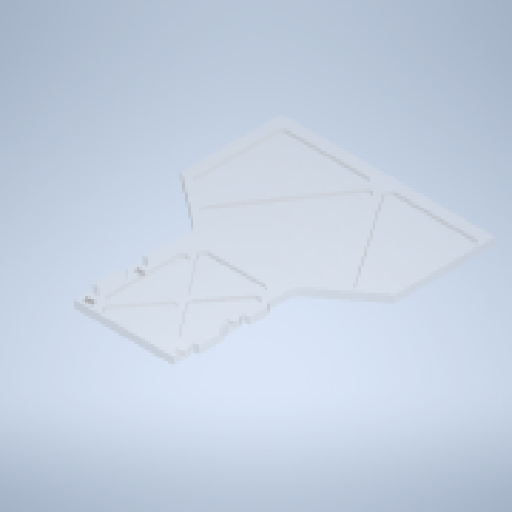
# Autodesk Inventor part: new_hera
Saved by Autodesk Inventor 2024 (Build 280153000, 153)
## iProperties
Created: 2023-12-17
Part Number: new_hera
Material: ポリカーボネート、クリア
Document SubType Name: Modeling
Designer: right
Density: 1.2 g/cm^3
Appearance: ポリカーボネート - クリア
Mass: 15.0866 g
Surface Area: 150.969 cm^2
Volume: 12.5721 cm^3
Author: right
Autodesk Inventor part; units mm, degrees
ref_plane "YZ Plane" through (0, 0, 0) normal (1, 0, 0) x (0, 1, 0)
ref_plane "XZ Plane" through (0, 0, 0) normal (0, 1, 0) x (-1, 0, 0)
ref_plane "XY Plane" through (0, 0, 0) normal (0, 0, 1) x (1, 0, 0)
sketch "スケッチ1" plane through (0, 0, 0) normal (0, 1, 0) x (-1, 0, 0)
  line L0 (-19.75, 24) -> (19.75, 24)
  line L1 (19.75, 24) -> (19.75, -24)
  line L2 (19.75, -24) -> (-19.75, -24)
  line L3 (-19.75, -24) -> (-19.75, 24)
  line L4 (-19.75, 24) -> (19.75, -24) construction
  line L5 (19.75, 24) -> (-19.75, -24) construction
  line L6 (19.75, 0) -> (-19.75, 0) construction
  line L7 (-19.75, 0) -> (19.75, -24) construction
  line L8 (19.75, 0) -> (-19.75, -24) construction
  line L9 (21.25, 15) -> (-21.25, 15)
  line L10 (-21.25, 15) -> (-21.25, 5)
  line L11 (-21.25, 5) -> (21.25, 5)
  line L12 (21.25, 5) -> (21.25, 15)
  line L13 (21.25, 15) -> (-21.25, 5) construction
  line L14 (-21.25, 15) -> (21.25, 5) construction
  circle A0 centre (19.75, 3.9) radius 1.1
  line L15 (0, 5) -> (0, 10) construction
  line L16 (21.25, 10) -> (0, 10) construction
  circle A1 centre (19.75, 16.1) radius 1.1
  circle A2 centre (-19.75, 3.9) radius 1.1
  circle A3 centre (-19.75, 16.1) radius 1.1
  line L17 (21.25, -15) -> (-21.25, -15)
  line L18 (-21.25, -15) -> (-21.25, -5)
  line L19 (-21.25, -5) -> (21.25, -5)
  line L20 (21.25, -5) -> (21.25, -15)
  line L21 (21.25, -15) -> (-21.25, -5) construction
  line L22 (-21.25, -15) -> (21.25, -5) construction
  circle A4 centre (19.75, -3.9) radius 1.1
  line L23 (0, -5) -> (0, -10) construction
  line L24 (21.25, -10) -> (0, -10) construction
  circle A5 centre (19.75, -16.1) radius 1.1
  circle A6 centre (-19.75, -16.1) radius 1.1
  circle A7 centre (-19.75, -3.9) radius 1.1
  point P0 (0, 0)
  point P1 (-19.75, 17.2)
  point P2 (-19.75, 15)
  point P3 (-19.75, 5)
  point P4 (-19.75, 2.8)
  point P5 (-19.75, -2.8)
  point P6 (-19.75, -5)
  point P7 (-19.75, -15)
  point P8 (-19.75, -17.2)
  point P9 (19.75, -17.2)
  point P10 (19.75, -15)
  point P11 (19.75, -5)
  point P12 (19.75, -2.8)
  point P13 (19.75, 2.8)
  point P14 (19.75, 5)
  point P15 (19.75, 15)
  point P16 (19.75, 17.2)
  point P17 (19.75, -15)
  point P18 (-19.75, -15)
  dimension "d1" = 48
  dimension "d2" = 39.5
  dimension "d3" = 10
  dimension "d4" = 1.5
  dimension "d5" = 2.2
  dimension "d6" = 10
  dimension "d7" = 1.5
  constraints: 50 end point, 14 symmetric about line, 8 centre point, 8 midpoint, 4 parallel, 3 perpendicular, 2 horizontal, 1 point on line, 1 tangent, 1 vertical, 7 other
  measures "d1" distance of L2.end L0.start
  measures "d2" distance between parallel lines of L3 L1
  measures "d3" distance of L10.end L9.end
  measures "d4" distance between parallel lines of L3 L10
  measures "d5" diameter of A0
  measures "d6" distance between parallel lines of L19 L11
  measures "d7" distance between parallel lines of L1 L12
extrude "押し出し1" add sketch "スケッチ1" along normal blind 3 contours L0 L1 A1 L9 A3 L3 | L9 L1 L11 L3 | L3 L11 L10 L9 | L9 L12 L11 L1 | L11 A0 L1 A4 L19 A7 L3 A2 | L19 L1 L17 L3 | L3 L17 L18 L19 | L19 L20 L17 L1 | A6 L3 | L17 A5 L1 L2 L3 A6 | L1 A5 picked at (-19.4196, -15.9409) picked at (19.6623, -16.456)
sketch "スケッチ2" plane through (-19.75, 0, 17.2) normal (-1, 0, 0) x (0, 0, 1)
  line L0 (6.8, 0) -> (6.8, 3) construction
  line L1 (6.8, 1.5) -> (-41.2, 1.5) construction
  line L2 (-41.2, 0) -> (-41.2, 3) construction
  line L3 (-2.2, 3) -> (-12.2, 3) construction
  line L4 (-7.2, 3) -> (-7.2, 0) construction
  line L5 (-12.2, 0) -> (-12.2, 3) construction
  point P0 (-17.2, 0)
  point P1 (-17.2, 1.5)
  point P2 (2.8, 1.5)
  dimension "d10" = 5
  constraints: 4 end point, 4 midpoint, 1 symmetric about line, 1 vertical
  measures "d10" distance from line of L5 point (-17.2, 1.5)
hole "穴1" at (-19.75, 1.5, 0) at (-19.75, 1.5, 20) direction (1, 0, 0) diameter 1.567 end through all thread size "M2x0.4" class "6H" standard "ISO Metric profile"
sketch "スケッチ3" plane through (0, 3, 0) normal (0, 1, 0) x (1, 0, 0)
  line L0 (42.5, 81.5) -> (-42.5, 81.5)
  line L1 (19.75, 24) -> (-19.75, 24) projected
  circle A0 centre (0, -173.5) radius 4 projected
  line L2 (0, 81.5) -> (0, 24) construction
  line L3 (42.5, 81.5) -> (42.5, 41.5)
  line L4 (42.5, 41.5) -> (19.75, 24)
  line L5 (-42.5, 41.5) -> (-19.75, 24)
  line L6 (-42.5, 81.5) -> (-42.5, 41.5)
  point P0 (0, 0)
  dimension "d18" = 255
  dimension "d19" = 85
  dimension "d20" = 40
  constraints: 12 end point, 2 midpoint, 2 vertical, 1 horizontal, 1 symmetric about line, 1 vertical alignment
  measures "d18" distance from line of A0.centre L0
  measures "d19" distance of L0.start L0.end
  measures "d20" distance of L0.start L3.end
extrude "押し出し2" add sketch "スケッチ3" against normal up to surface (3 mm away) contours L3 L4 L1 L5 L6 L0
fillet "フィレット1" radius 5.75 2 edges at (-19.75, 1.5, -24) (19.75, 1.5, -24)
sketch "スケッチ6" plane through (0, 3, 0) normal (0, 1, 0) x (1, 0, 0)
  arc A0 (19.75, 15) -> (21.3608, 12.8804) centre (21.95, 15) ccw
  line L0 (19.75, 15) -> (19.75, 21.1687) projected
  line L1 (21.25, 14) -> (21.25, -21.2075)
  line L2 (21.25, 18) -> (21.25, 14)
  line L3 (21.25, 15) -> (19.75, 15) projected
  line L4 (0, 0) -> (0, -24) construction
  line L5 (-19.75, -24) -> (19.75, -24) construction
  arc A1 (-21.3608, 12.8804) -> (-19.75, 15) centre (-21.95, 15) ccw
  line L6 (-21.25, 15) -> (-19.75, 15)
  line L7 (-21.25, 14) -> (-21.25, 18)
  line L8 (-21.25, 14) -> (-21.25, -21.2075)
  point P0 (21.25, 12.9143)
  point P1 (-21.25, 12.9143)
  dimension "d30" = 2.2
  constraints: 12 end point, 5 symmetric about line, 4 point on circle, 4 vertical, 2 centre point, 1 midpoint, 1 tangent, 7 other
  measures "d30" radius of A0
extrude "押し出し4" cut sketch "スケッチ6" against normal through all
sketch "スケッチ7" plane through (0, 0, 0) normal (0, -1, 0) x (1, 0, 0)
  line L0 (-19.75, -21.1687) -> (-19.75, -15) projected
  line L1 (19.75, -15) -> (19.75, -21.1687) projected
  line L2 (-19.75, -15) -> (19.75, -15)
  line L3 (-21.9942, -25.7263) -> (-42.5, -41.5) projected
  arc A0 (-21.9942, -25.7263) -> (-19.75, -21.1687) centre (-25.5, -21.1687) ccw projected
  line L4 (-42.5, -41.5) -> (-42.5, -81.5) projected
  line L5 (-42.5, -81.5) -> (42.5, -81.5) projected
  arc A1 (19.75, -21.1687) -> (21.9942, -25.7263) centre (25.5, -21.1687) ccw projected
  line L6 (42.5, -41.5) -> (21.9942, -25.7263) projected
  line L7 (42.5, -81.5) -> (42.5, -41.5) projected
  line L8 (-16.75, -21.1687) -> (-16.75, -18)
  line L9 (-16.75, -18) -> (16.75, -18)
  line L10 (16.75, -18) -> (16.75, -21.1687)
  arc A2 (16.75, -21.1687) -> (20.165, -28.1042) centre (25.5, -21.1687) ccw
  line L11 (20.165, -28.1042) -> (39.5, -42.9772)
  line L12 (39.5, -42.9772) -> (39.5, -78.5)
  line L13 (39.5, -78.5) -> (-39.5, -78.5)
  line L14 (-39.5, -78.5) -> (-39.5, -42.9772)
  line L15 (-39.5, -42.9772) -> (-20.165, -28.1042)
  arc A3 (-20.165, -28.1042) -> (-16.75, -21.1687) centre (-25.5, -21.1687) ccw
  line L16 (0, -78.5) -> (-29.8325, -35.5407) construction
  line L17 (0, -78.5) -> (29.8325, -35.5407) construction
  line L18 (0, -78.5) -> (0, -18) construction
  line L19 (1.1903, -77.5843) -> (-28.5587, -34.7452)
  line L20 (-28.5587, -34.7452) -> (-31.0229, -36.4563)
  line L21 (-31.0229, -36.4563) -> (-1.2738, -79.2955)
  line L22 (-1.2738, -79.2955) -> (1.1903, -77.5843)
  line L23 (1.1903, -77.5843) -> (-31.0229, -36.4563) construction
  line L24 (-28.5587, -34.7452) -> (-1.2738, -79.2955) construction
  line L25 (-1.1903, -77.5843) -> (28.6422, -34.625)
  line L26 (31.0229, -36.4563) -> (1.2738, -79.2955)
  line L27 (20.165, -28.1042) -> (-20.165, -28.1042)
  line L28 (-20.165, -28.1042) -> (-20.165, -25.1042)
  line L29 (-20.165, -25.1042) -> (20.165, -25.1042)
  line L30 (20.165, -25.1042) -> (20.165, -28.1042)
  line L31 (-28.5587, -34.7452) -> (-28.6355, -34.6199)
  point P0 (0, 0)
  point P1 (-14.9163, -57.0203)
  point P2 (28.5587, -34.7452)
  point P3 (31.0229, -36.4563)
  point P4 (-29.2396, -35.4437)
  point P5 (-1.8262, -78.5)
  point P6 (-31.7065, -37.1534)
  point P7 (0, -75.8702)
  point P8 (29.2396, -35.4437)
  point P9 (1.8262, -78.5)
  point P10 (-17.685, -25.1042)
  point P11 (17.685, -25.1042)
  point P12 (-0.1282, -78.5)
  point P13 (-19.5553, -28.8968)
  point P14 (-19.5553, -28.8968)
  dimension "d33" = 3
  dimension "d34" = 3
  dimension "d38" = 3
  constraints: 50 end point, 8 point on line, 7 midpoint, 5 parallel, 4 point on circle, 4 symmetric about line, 2 centre point, 2 horizontal, 2 perpendicular, 9 other
  measures "d33" radial gap between concentric circles of A0 A3
  measures "d34" distance of L20.end L19.end
  measures "d38" distance between parallel lines of L27 L29
extrude "押し出し5" cut sketch "スケッチ7" against normal blind 1.5 contours L27 L11 L25 L19 L31 L15 | L21 L13 L14 L15 | L11 L12 L13 L26
fillet "フィレット3" radius 2 14 edges at (0, 0.75, -75.8702) (1.8262, 0.75, -78.5) (-1.8262, 0.75, -78.5) (31.0229, 0.75, -36.4563) (39.5, 0.75, -78.5) (39.5, 0.75, -42.9772) (-39.5, 0.75, -42.9772) (-39.5, 0.75, -78.5) (-31.0229, 0.75, -36.4563) (-20.165, 0.75, -28.1042) (20.165, 0.75, -28.1042) (28.6422, 0.75, -34.625) (-28.6355, 0.75, -34.6199) (-28.5587, 0.75, -34.7452)
sketch "スケッチ8" plane through (0, 0, 0) normal (0, -1, 0) x (1, 0, 0)
  line L0 (19.75, 20.7835) -> (-19.75, 20.7835) projected
  line L1 (-10.771, -20.7835) -> (10.771, -20.7835)
  line L2 (16.25, -13.479) -> (16.25, 13.479)
  line L3 (10.771, 20.7835) -> (-10.771, 20.7835)
  line L4 (-16.25, 13.479) -> (-16.25, -13.479)
  line L5 (-16.25, -20.7835) -> (16.25, 20.7835) construction
  line L6 (16.25, -20.7835) -> (-16.25, 20.7835) construction
  line L7 (-21.25, 5) -> (-21.25, 15) projected
  arc A0 (-14.25, 20.7835) -> (-16.25, 18.7835) centre (-14.25, 18.7835) ccw
  arc A1 (16.25, 18.7835) -> (14.25, 20.7835) centre (14.25, 18.7835) ccw
  arc A2 (14.25, -20.7835) -> (16.25, -18.7835) centre (14.25, -18.7835) ccw
  arc A3 (-16.25, -18.7835) -> (-14.25, -20.7835) centre (-14.25, -18.7835) ccw
  line L8 (12.3514, -17.5578) -> (-12.6696, 14.7046)
  line L9 (-16.4544, 19.5849) -> (-14.874, 20.8106)
  line L10 (-12.3514, 17.5578) -> (12.6696, -14.7046)
  line L11 (16.4544, -19.5849) -> (14.874, -20.8106)
  line L12 (14.874, -20.8106) -> (-14.874, 20.8106) construction
  line L13 (-16.4544, 19.5849) -> (16.4544, -19.5849) construction
  arc A4 (-12.6696, 14.7046) -> (-16.25, 13.479) centre (-14.25, 13.479) ccw
  arc A5 (-10.771, 20.7835) -> (-12.3514, 17.5578) centre (-10.771, 18.7835) ccw
  arc A6 (12.6696, -14.7046) -> (16.25, -13.479) centre (14.25, -13.479) ccw
  arc A7 (10.771, -20.7835) -> (12.3514, -17.5578) centre (10.771, -18.7835) ccw
  line L14 (0, 0) -> (0, 20.7835) construction
  line L15 (-12.3514, -17.5578) -> (12.6696, 14.7046)
  line L16 (12.3514, 17.5578) -> (-12.6696, -14.7046)
  arc A8 (12.3514, 17.5578) -> (10.771, 20.7835) centre (10.771, 18.7835) ccw
  arc A9 (16.25, 13.479) -> (12.6696, 14.7046) centre (14.25, 13.479) ccw
  arc A10 (-12.3514, -17.5578) -> (-10.771, -20.7835) centre (-10.771, -18.7835) ccw
  arc A11 (-16.25, -13.479) -> (-12.6696, -14.7046) centre (-14.25, -13.479) ccw
  point P0 (-15.6642, 20.1977)
  point P1 (12.6696, 14.7046)
  point P2 (12.3514, 17.5578)
  point P3 (-12.6696, -14.7046)
  point P4 (-12.3514, -17.5578)
  point P5 (0, 1.6317)
  point P6 (1.2655, 0)
  point P7 (0, -1.6317)
  point P8 (-1.2655, 0)
  dimension "d39" = 5
  dimension "d40" = 2
  dimension "d41" = 2
  dimension "d42" = 2
  dimension "d43" = 2
  constraints: 30 end point, 25 point on circle, 25 point on line, 24 tangent, 12 centre point, 9 equal radius, 6 midpoint, 4 parallel, 4 symmetric about line, 3 perpendicular, 1 horizontal
  measures "d39" distance between parallel lines of L7 L4
  measures "d40" radius of A0
  measures "d41" distance between parallel lines of L8 L10
  measures "d42" radius of A4
  measures "d43" radius of A8
extrude "押し出し6" cut sketch "スケッチ8" against normal blind 1.5 contours A8 L16 L10 A5 L0 | L15 A9 L2 A6 L10 | L8 A7 L1 A10 L15 | L16 A11 L4 A4 L8
sketch "スケッチ9" plane through (0, 1.5, 0) normal (0, -1, 0) x (1, 0, 0)
  line L0 (12.6696, -14.7046) -> (1.2655, 0) projected
  line L1 (1.2655, 0) -> (12.6696, 14.7046) projected
  arc A0 (16.25, 13.479) -> (12.6696, 14.7046) centre (14.25, 13.479) ccw projected
  line L2 (16.25, 13.479) -> (16.25, -13.479) projected
  arc A1 (12.6696, -14.7046) -> (16.25, -13.479) centre (14.25, -13.479) ccw projected
  line L3 (-12.3514, -17.5578) -> (0, -1.6317) projected
  line L4 (0, -1.6317) -> (12.3514, -17.5578) projected
  arc A2 (10.771, -20.7835) -> (12.3514, -17.5578) centre (10.771, -18.7835) ccw projected
  line L5 (10.771, -20.7835) -> (-10.771, -20.7835) projected
  arc A3 (-12.3514, -17.5578) -> (-10.771, -20.7835) centre (-10.771, -18.7835) ccw projected
  arc A4 (-10.771, 20.7835) -> (-12.3514, 17.5578) centre (-10.771, 18.7835) ccw projected
  line L6 (-10.771, 20.7835) -> (10.771, 20.7835) projected
  arc A5 (12.3514, 17.5578) -> (10.771, 20.7835) centre (10.771, 18.7835) ccw projected
  line L7 (12.3514, 17.5578) -> (0, 1.6317) projected
  line L8 (0, 1.6317) -> (-12.3514, 17.5578) projected
  line L9 (-12.6696, 14.7046) -> (-1.2655, 0) projected
  line L10 (-1.2655, 0) -> (-12.6696, -14.7046) projected
  arc A6 (-16.25, -13.479) -> (-12.6696, -14.7046) centre (-14.25, -13.479) ccw projected
  line L11 (-16.25, -13.479) -> (-16.25, 13.479) projected
  arc A7 (-12.6696, 14.7046) -> (-16.25, 13.479) centre (-14.25, 13.479) ccw projected
  line L12 (-29.8251, -38.1811) -> (-4.0073, -75.3592) projected
  arc A8 (-5.65, -78.5) -> (-4.0073, -75.3592) centre (-5.65, -76.5) ccw projected
  line L13 (-5.65, -78.5) -> (-37.5, -78.5) projected
  arc A9 (-39.5, -76.5) -> (-37.5, -78.5) centre (-37.5, -76.5) ccw projected
  line L14 (-39.5, -76.5) -> (-39.5, -43.962) projected
  arc A10 (-38.7194, -42.3768) -> (-39.5, -43.962) centre (-37.5, -43.962) ccw projected
  line L15 (-38.7194, -42.3768) -> (-32.6873, -37.7366) projected
  arc A11 (-29.8251, -38.1811) -> (-32.6873, -37.7366) centre (-31.4679, -39.3219) ccw projected
  line L16 (4.0073, -75.3592) -> (29.8251, -38.1811) projected
  arc A12 (32.6873, -37.7366) -> (29.8251, -38.1811) centre (31.4679, -39.3219) ccw projected
  line L17 (32.6873, -37.7366) -> (38.7194, -42.3768) projected
  arc A13 (39.5, -43.962) -> (38.7194, -42.3768) centre (37.5, -43.962) ccw projected
  line L18 (39.5, -43.962) -> (39.5, -76.5) projected
  arc A14 (37.5, -78.5) -> (39.5, -76.5) centre (37.5, -76.5) ccw projected
  line L19 (37.5, -78.5) -> (5.65, -78.5) projected
  arc A15 (4.0073, -75.3592) -> (5.65, -78.5) centre (5.65, -76.5) ccw projected
  line L20 (-27.1323, -33.4636) -> (-20.7042, -28.5189) projected
  arc A16 (-19.4848, -28.1042) -> (-20.7042, -28.5189) centre (-19.4848, -30.1042) ccw projected
  line L21 (-19.4848, -28.1042) -> (19.4848, -28.1042) projected
  arc A17 (20.7042, -28.5189) -> (19.4848, -28.1042) centre (19.4848, -30.1042) ccw projected
  line L22 (20.7042, -28.5189) -> (27.1323, -33.4636) projected
  arc A18 (27.5556, -36.1896) -> (27.1323, -33.4636) centre (25.9129, -35.0489) ccw projected
  line L23 (27.5556, -36.1896) -> (1.6427, -73.5046) projected
  arc A19 (-1.6427, -73.5046) -> (1.6427, -73.5046) centre (0, -72.3639) ccw projected
  line L24 (-1.6427, -73.5046) -> (-27.5556, -36.1896) projected
  arc A20 (-27.1323, -33.4636) -> (-27.5556, -36.1896) centre (-25.9129, -35.0489) ccw projected
  arc A21 (21.25, -12.9143) -> (19.75, -15) centre (21.95, -15) ccw projected
  line L25 (21.25, -5) -> (21.25, -12.9143) projected
  line L26 (19.75, -5) -> (21.25, -5) projected
  arc A22 (19.75, -2.8) -> (19.75, -5) centre (19.75, -3.9) ccw projected
  line L27 (19.75, 2.8) -> (19.75, -2.8) projected
  arc A23 (19.75, 5) -> (19.75, 2.8) centre (19.75, 3.9) ccw projected
  line L28 (21.25, 5) -> (19.75, 5) projected
  line L29 (21.25, 15) -> (21.25, 5) projected
  line L30 (19.75, 15) -> (21.25, 15) projected
  arc A24 (19.75, 17.2) -> (19.75, 15) centre (19.75, 16.1) ccw projected
  line L31 (19.75, 24) -> (19.75, 17.2) projected
  line L32 (-19.75, 24) -> (19.75, 24) projected
  line L33 (-19.75, 17.2) -> (-19.75, 24) projected
  arc A25 (-19.75, 15) -> (-19.75, 17.2) centre (-19.75, 16.1) ccw projected
  line L34 (-21.25, 15) -> (-19.75, 15) projected
  line L35 (-21.25, 5) -> (-21.25, 15) projected
  line L36 (-19.75, 5) -> (-21.25, 5) projected
  arc A26 (-19.75, 2.8) -> (-19.75, 5) centre (-19.75, 3.9) ccw projected
  line L37 (-19.75, -2.8) -> (-19.75, 2.8) projected
  arc A27 (-19.75, -5) -> (-19.75, -2.8) centre (-19.75, -3.9) ccw projected
  line L38 (-21.25, -5) -> (-19.75, -5) projected
  line L39 (-21.25, -12.9143) -> (-21.25, -5) projected
  arc A28 (-19.75, -15) -> (-21.25, -12.9143) centre (-21.95, -15) ccw projected
  line L40 (-19.75, -21.1687) -> (-19.75, -15) projected
  arc A29 (-21.9942, -25.7263) -> (-19.75, -21.1687) centre (-25.5, -21.1687) ccw projected
  line L41 (-21.9942, -25.7263) -> (-42.5, -41.5) projected
  line L42 (-42.5, -41.5) -> (-42.5, -81.5) projected
  line L43 (-42.5, -81.5) -> (42.5, -81.5) projected
  line L44 (42.5, -81.5) -> (42.5, -41.5) projected
  line L45 (42.5, -41.5) -> (21.9942, -25.7263) projected
  arc A30 (19.75, -21.1687) -> (21.9942, -25.7263) centre (25.5, -21.1687) ccw projected
  line L46 (19.75, -15) -> (19.75, -21.1687) projected
  line L47 (19.75, 20.7835) -> (-19.75, 20.7835) projected
  line L48 (16.25, -20.7835) -> (-16.25, -20.7835)
  line L49 (-16.25, -20.7835) -> (-16.25, 20.7835)
  line L50 (-16.25, 20.7835) -> (16.25, 20.7835)
  line L51 (16.25, 20.7835) -> (16.25, -20.7835)
  line L52 (16.25, -20.7835) -> (-16.25, 20.7835) construction
  line L53 (-16.25, -20.7835) -> (16.25, 20.7835) construction
  point P0 (0, 0)
  point P1 (-10.771, -20.7835)
  constraints: 12 end point, 2 midpoint, 2 parallel, 1 horizontal, 1 perpendicular, 1 point on line, 1 vertical alignment
extrude "押し出し7" add sketch "スケッチ9" against normal blind 1.5 contours A1 L51 L48 A2 L4 L3 A3 L49 A6 L10 L9 A7 L47 A4 L8 L7 A5 A0 L1 L0 | L0 L1 A0 L2 A1 | L47 L6 L33 L32 L31 | L5 A3 L3 L4 A2 | A5 L7 L8 A4 L6 | L11 A7 L9 L10 A6
extrude "押し出し8" add sketch "スケッチ9" along normal blind 1.5 contours A1 L51 L48 A2 L4 L3 A3 L49 A6 L10 L9 A7 L47 A4 L8 L7 A5 A0 L1 L0
fillet "フィレット4" radius 2 4 edges at (1.2655, 0.75, 0) (0, 0.75, 1.6317) (-1.2655, 0.75, 0) (0, 0.75, -1.6317)
